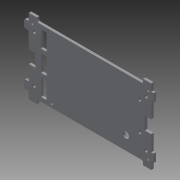
# Autodesk Inventor part: Main Platform 25100813
Saved by Autodesk Inventor 2015 (Build 190159000, 159)
## iProperties
Created: 2013-05-24
Part Number: Main Platform 25100813
Material: Generic
Document SubType Name: Modeling
Designer: Eric
Density: 1 g/cm^3
Appearance: Default
Author: Eric
Autodesk Inventor part; units mm, degrees
ref_plane "YZ Plane" through (0, 0, 0) normal (1, 0, 0) x (0, 1, 0)
ref_plane "XZ Plane" through (0, 0, 0) normal (0, 1, 0) x (-1, 0, 0)
ref_plane "XY Plane" through (0, 0, 0) normal (0, 0, 1) x (1, 0, 0)
sketch "Sketch1" plane through (0, 0, 0) normal (0, 1, 0) x (-1, 0, 0)
  line L0 (-77, 37.5) -> (-80, 37.5)
  line L1 (-80, 27.5) -> (-77, 27.5)
  line L2 (-77, 27.5) -> (-77, 8)
  line L3 (-77, 8) -> (-69, 8)
  line L4 (-77, -37.5) -> (-80, -37.5)
  line L5 (-80, -27.5) -> (-77, -27.5)
  line L6 (-77, -27.5) -> (-77, -8)
  line L7 (-77, -8) -> (-69, -8)
  line L8 (-69, -8) -> (-69, 8)
  line L9 (-80, 37.5) -> (-80, 27.5)
  line L10 (-80, -37.5) -> (-80, -27.5)
  line L11 (75, 37.5) -> (79, 37.5)
  line L12 (81, 35.5) -> (81, 29.5)
  line L13 (79, 27.5) -> (75, 27.5)
  line L14 (75, -37.5) -> (79, -37.5)
  line L15 (81, -35.5) -> (81, -29.5)
  line L16 (79, -27.5) -> (75, -27.5)
  line L17 (75, 46.5) -> (75, 37.5)
  line L18 (75, -37.5) -> (75, -46.5)
  line L19 (-77, 37.5) -> (-77, 46.5)
  line L20 (-77, -46.5) -> (-77, -37.5)
  arc A0 (81, 35.5) -> (79, 37.5) centre (79, 35.5) ccw
  arc A1 (79, 27.5) -> (81, 29.5) centre (79, 29.5) ccw
  arc A2 (81, -29.5) -> (79, -27.5) centre (79, -29.5) ccw
  arc A3 (79, -37.5) -> (81, -35.5) centre (79, -35.5) ccw
  line L21 (75, 7.5) -> (67, 7.5)
  line L22 (67, 7.5) -> (67, -8.5)
  line L23 (67, -8.5) -> (75, -8.5)
  line L24 (75, 27.5) -> (75, 7.5)
  line L25 (75, -8.5) -> (75, -27.5)
  line L26 (-67, 46.5) -> (-67, 43.5)
  line L27 (-65, 41.5) -> (63, 41.5)
  line L28 (65, 43.5) -> (65, 46.5)
  line L29 (-77, 46.5) -> (-67, 46.5)
  line L30 (65, 46.5) -> (75, 46.5)
  line L31 (-67, -46.5) -> (-67, -43.5)
  line L32 (-65, -41.5) -> (63, -41.5)
  line L33 (65, -43.5) -> (65, -46.5)
  line L34 (-77, -46.5) -> (-67, -46.5)
  line L35 (65, -46.5) -> (75, -46.5)
  arc A4 (65, -43.5) -> (63, -41.5) centre (63, -43.5) ccw
  arc A5 (-65, -41.5) -> (-67, -43.5) centre (-65, -43.5) ccw
  arc A6 (-67, 43.5) -> (-65, 41.5) centre (-65, 43.5) ccw
  arc A7 (63, 41.5) -> (65, 43.5) centre (63, 43.5) ccw
  point P0 (0, 0)
  point P1 (81, 37.5)
  point P2 (81, 27.5)
  point P3 (81, -37.5)
  point P4 (81, -27.5)
  point P5 (-67, 41.5)
  point P6 (-67, -41.5)
  dimension "d5" = 10
  dimension "d20" = 3
  dimension "d43" = 3
  dimension "d44" = 8
  dimension "d49" = 10
  dimension "d50" = 10
  dimension "d53" = 6
  dimension "d54" = 6
  dimension "d74" = 2
  dimension "d75" = 8
  dimension "d76" = 8
  dimension "d77" = 16
  dimension "d89" = 8
  dimension "d113" = 5
  dimension "d114" = 10
  dimension "d115" = 10
  dimension "d116" = 5
  dimension "d117" = 10
  dimension "d118" = 10
  dimension "d119" = 2
  dimension "d120" = 6
  dimension "d124" = 41.5
  dimension "d127" = 6
  dimension "d128" = 80
  dimension "d129" = 3
  dimension "d130" = 132
  dimension "d133" = 3
  dimension "d135" = 33
  dimension "d136" = 93
  dimension "d140" = 16
  dimension "d142" = 8
  dimension "d144" = 10
  dimension "d145" = 5
  dimension "d146" = 5
  dimension "d147" = 27.5
  dimension "d148" = 27.5
  dimension "d149" = 27.5
  dimension "d150" = 27.5
  dimension "d164" = 161
  constraints: 72 end point, 37 perpendicular, 16 point on circle, 16 tangent, 12 point on line, 10 parallel, 8 centre point, 6 equal radius, 2 collinear, 2 horizontal
  measures "d5" distance between parallel lines of L1 L0
  measures "d20" distance of L5.start L5.end
  measures "d43" distance of L1.start L1.end
  measures "d44" distance of L2.end L3.end
  measures "d49" distance between parallel lines of L13 L11
  measures "d50" distance between parallel lines of L14 L16
  measures "d53" distance of L11.start point (81, 37.5)
  measures "d54" distance of L14.start point (81, -37.5)
  measures "d74" radius of A0
  measures "d75" distance of L21.start L21.end
  measures "d76" distance of L22.end L23.end
  measures "d77" distance between parallel lines of L23 L21
  measures "d89" distance of L6.end L7.end
  measures "d113" distance of L26.start point (-67, 41.5)
  measures "d114" distance between parallel lines of L19 L26
  measures "d115" distance between parallel lines of L17 L28
  measures "d116" distance of L31.start point (-67, -41.5)
  measures "d117" distance between parallel lines of L20 L31
  measures "d118" distance between parallel lines of L33 L18
  measures "d119" radius of A4
  measures "d120" distance between parallel lines of L24 L12
  measures "d124" distance from line of L27 point (0, 0)
  measures "d127" distance between parallel lines of L25 L15
  measures "d128" distance from line of point (0, 0) L9
  measures "d129" distance of L0.start L0.end
  measures "d130" distance between parallel lines of L28 L26
  measures "d133" distance of L4.start L4.end
  measures "d135" distance between parallel lines of L32 L23
  measures "d136" distance between parallel lines of L34 L29
  measures "d140" distance of L7.end L3.end
  measures "d142" distance from line of point (0, 0) L3
  measures "d144" distance between parallel lines of L5 L4
  measures "d145" distance between parallel lines of L30 L27
  measures "d146" distance between parallel lines of L35 L32
  measures "d147" distance from line of point (0, 0) L1
  measures "d148" distance from line of point (0, 0) L5
  measures "d149" distance from line of point (0, 0) L16
  measures "d150" distance from line of point (0, 0) L13
  measures "d164" distance between parallel lines of L12 L9
extrude "Extrusion1" add sketch "Sketch1" along normal blind 3
sketch "Sketch2" plane through (0, 0, 0) normal (0, -1, 0) x (1, 0, 0)
  line L0 (77, 46.5) -> (77, 37.5) projected
  line L1 (-75, 7.5) -> (-75, 27.5) projected
  line L2 (-75, -27.5) -> (-75, -8.5) projected
  line L3 (-70, 30.5) -> (-67, 30.5)
  line L4 (-67, 30.5) -> (-67, 27.5)
  line L5 (-67, 27.5) -> (-70, 27.5)
  line L6 (-70, 27.5) -> (-70, 30.5)
  line L7 (-70, -27.5) -> (-67, -27.5)
  line L8 (-67, -27.5) -> (-67, -30.5)
  line L9 (-67, -30.5) -> (-70, -30.5)
  line L10 (-70, -30.5) -> (-70, -27.5)
  line L11 (77, -37.5) -> (77, -46.5) projected
  line L12 (69, 27.5) -> (72, 27.5)
  line L13 (72, 27.5) -> (72, 30.5)
  line L14 (72, 30.5) -> (69, 30.5)
  line L15 (69, 30.5) -> (69, 27.5)
  line L16 (69, -30.5) -> (72, -30.5)
  line L17 (72, -30.5) -> (72, -27.5)
  line L18 (72, -27.5) -> (69, -27.5)
  line L19 (69, -27.5) -> (69, -30.5)
  line L20 (77, -8) -> (77, -27.5) projected
  line L21 (77, 27.5) -> (77, 8) projected
  line L22 (61, 25) -> (64, 25)
  line L23 (64, 25) -> (64, 20)
  line L24 (64, 20) -> (61, 20)
  line L25 (61, 20) -> (61, 25)
  line L26 (61, -10) -> (64, -10)
  line L27 (64, -10) -> (64, -15)
  line L28 (64, -15) -> (61, -15)
  line L29 (61, -15) -> (61, -10)
  line L30 (65, -41.5) -> (-63, -41.5) projected
  point P0 (0, 0)
  dimension "d79" = 3
  dimension "d80" = 3
  dimension "d81" = 3
  dimension "d82" = 3
  dimension "d83" = 5
  dimension "d84" = 5
  dimension "d85" = 27.5
  dimension "d86" = 27.5
  dimension "d90" = 5
  dimension "d91" = 5
  dimension "d92" = 27.5
  dimension "d93" = 27.5
  dimension "d94" = 3
  dimension "d95" = 3
  dimension "d96" = 3
  dimension "d97" = 3
  dimension "d151" = 5
  dimension "d152" = 3
  dimension "d153" = 5
  dimension "d154" = 3
  dimension "d155" = 30
  dimension "d161" = 16
  dimension "d162" = 16
  dimension "d165" = 31.5
  constraints: 48 end point, 12 parallel, 6 horizontal, 6 perpendicular
  measures "d79" distance of L5.end L3.start
  measures "d80" distance of L3.start L3.end
  measures "d81" distance of L9.end L7.start
  measures "d82" distance of L8.end L9.end
  measures "d83" distance between parallel lines of L2 L10
  measures "d84" distance between parallel lines of L1 L6
  measures "d85" distance from line of point (0, 0) L7
  measures "d86" distance from line of point (0, 0) L5
  measures "d90" distance between parallel lines of L0 L13
  measures "d91" distance between parallel lines of L11 L17
  measures "d92" distance from line of point (0, 0) L18
  measures "d93" distance from line of point (0, 0) L12
  measures "d94" distance of L14.end L12.start
  measures "d95" distance of L12.start L12.end
  measures "d96" distance of L17.end L18.end
  measures "d97" distance of L16.end L17.end
  measures "d151" distance of L24.end L22.start
  measures "d152" distance of L23.end L24.end
  measures "d153" distance of L28.end L26.start
  measures "d154" distance of L26.start L26.end
  measures "d155" distance between parallel lines of L26 L24
  measures "d161" distance between parallel lines of L21 L25
  measures "d162" distance between parallel lines of L20 L29
  measures "d165" distance from line of L30 L26.start
extrude "Extrusion5" cut sketch "Sketch2" against normal through all
sketch "Sketch4" plane through (0, 0, 0) normal (0, -1, 0) x (1, 0, 0)
  line L0 (-63, 41.5) -> (65, 41.5) projected
  line L1 (-75, 37.5) -> (-75, 46.5) projected
  line L2 (65, -41.5) -> (-63, -41.5) projected
  line L3 (77, -8) -> (77, -27.5) projected
  circle A0 centre (45.5, -24.5) radius 4
  circle A1 centre (73, 37) radius 1.5
  circle A2 centre (-71, 37) radius 1.5
  circle A3 centre (73, -37) radius 1.5
  line L4 (-75, 7.5) -> (-75, 27.5) projected
  line L5 (-75, -27.5) -> (-75, -8.5) projected
  line L6 (-59, 36.5) -> (-54, 36.5)
  line L7 (-53, 35.5) -> (-53, 16.5)
  line L8 (-54, 15.5) -> (-59, 15.5)
  line L9 (-60, 16.5) -> (-60, 35.5)
  line L10 (-59, 10.5) -> (-54, 10.5)
  line L11 (-53, 9.5) -> (-53, -9.5)
  line L12 (-54, -10.5) -> (-59, -10.5)
  line L13 (-60, -9.5) -> (-60, 9.5)
  line L14 (-59, -15.5) -> (-54, -15.5)
  line L15 (-53, -16.5) -> (-53, -35.5)
  line L16 (-54, -36.5) -> (-59, -36.5)
  line L17 (-60, -35.5) -> (-60, -16.5)
  arc A4 (-59, 36.5) -> (-60, 35.5) centre (-59, 35.5) ccw
  arc A5 (-53, 35.5) -> (-54, 36.5) centre (-54, 35.5) ccw
  arc A6 (-54, 15.5) -> (-53, 16.5) centre (-54, 16.5) ccw
  arc A7 (-60, 16.5) -> (-59, 15.5) centre (-59, 16.5) ccw
  arc A8 (-59, 10.5) -> (-60, 9.5) centre (-59, 9.5) ccw
  arc A9 (-53, 9.5) -> (-54, 10.5) centre (-54, 9.5) ccw
  arc A10 (-54, -10.5) -> (-53, -9.5) centre (-54, -9.5) ccw
  arc A11 (-60, -9.5) -> (-59, -10.5) centre (-59, -9.5) ccw
  arc A12 (-59, -15.5) -> (-60, -16.5) centre (-59, -16.5) ccw
  arc A13 (-53, -16.5) -> (-54, -15.5) centre (-54, -16.5) ccw
  arc A14 (-54, -36.5) -> (-53, -35.5) centre (-54, -35.5) ccw
  arc A15 (-60, -35.5) -> (-59, -36.5) centre (-59, -35.5) ccw
  circle A16 centre (-47, -37) radius 1.5
  point P0 (0, 0)
  point P1 (-53, 15.5)
  point P2 (-53, 36.5)
  point P3 (-60, 15.5)
  point P4 (-53, -10.5)
  point P5 (-53, 10.5)
  point P6 (-60, -10.5)
  point P7 (-53, -36.5)
  point P8 (-53, -15.5)
  point P9 (-60, -36.5)
  dimension "d167" = 17
  dimension "d168" = 8
  dimension "d169" = 3
  dimension "d170" = 3
  dimension "d171" = 144
  dimension "d172" = 4
  dimension "d173" = 31.5
  dimension "d176" = 3
  dimension "d177" = 74
  dimension "d179" = 4.5
  dimension "d181" = 4.5
  dimension "d184" = 4.5
  dimension "d185" = 21
  dimension "d186" = 7
  dimension "d187" = 15
  dimension "d188" = 5
  dimension "d189" = 21
  dimension "d190" = 7
  dimension "d191" = 5
  dimension "d192" = 15
  dimension "d193" = 21
  dimension "d194" = 5
  dimension "d195" = 15
  dimension "d196" = 7
  dimension "d197" = 1
  dimension "d200" = 3
  dimension "d201" = 4.5
  dimension "d202" = 24
  constraints: 24 end point, 24 point on circle, 24 tangent, 18 point on line, 17 centre point, 11 equal radius, 6 parallel, 3 horizontal, 3 perpendicular
  measures "d167" distance from line of L2 A0.centre
  measures "d168" diameter of A0
  measures "d169" diameter of A1
  measures "d170" diameter of A2
  measures "d171" distance of A1.centre A2.centre
  measures "d172" distance from line of L1 A2.centre
  measures "d173" distance from line of L3 A0.centre
  measures "d176" diameter of A3
  measures "d177" distance of A1.centre A3.centre
  measures "d179" distance from line of L0 A2.centre
  measures "d181" distance from line of A3.centre L2
  measures "d184" distance from line of A1.centre L0
  measures "d185" distance of point (-53, 36.5) point (-53, 15.5)
  measures "d186" distance of point (-53, 15.5) point (-60, 15.5)
  measures "d187" distance between parallel lines of L4 L9
  measures "d188" distance between parallel lines of L6 L0
  measures "d189" distance of point (-53, 10.5) point (-53, -10.5)
  measures "d190" distance of point (-53, -10.5) point (-60, -10.5)
  measures "d191" distance between parallel lines of L8 L10
  measures "d192" distance between parallel lines of L4 L13
  measures "d193" distance of point (-53, -15.5) point (-53, -36.5)
  measures "d194" distance between parallel lines of L12 L14
  measures "d195" distance between parallel lines of L17 L5
  measures "d196" distance of point (-53, -36.5) point (-60, -36.5)
  measures "d197" radius of A4
  measures "d200" diameter of A16
  measures "d201" distance from line of L2 A16.centre
  measures "d202" horizontal distance of A2.centre A16.centre
extrude "Extrusion8" cut sketch "Sketch4" against normal blind 10
body "Solid1"
